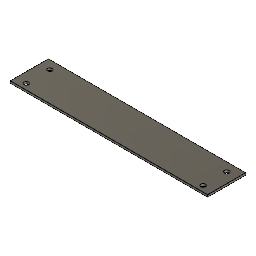
smmb_front-top (Autodesk Fusion 360 design; units mm, degrees)
Autodesk Fusion 360 part; units mm, degrees
sketch "Sketch1" plane through (0, 0, 0) normal (0, 0, 1) x (1, 0, 0)
  line L0 (0, 0) -> (134, 0)
  line L1 (134, 0) -> (134, 26)
  line L2 (134, 26) -> (0, 26)
  line L3 (0, 26) -> (0, 0)
  circle A0 centre (7, 20) radius 1.55
  circle A1 centre (7, 4) radius 1.55
  circle A2 centre (127, 20) radius 1.55
  circle A3 centre (127, 4) radius 1.55
  dimension "d1" = 134
  dimension "d2" = 26
  dimension "d3" = 3.1
  dimension "d4" = 7
  dimension "d5" = 6
  dimension "d6" = 3.1
  dimension "d7" = 7
  dimension "d8" = 4
  dimension "d9" = 3.1
  dimension "d10" = 3.1
  dimension "d11" = 7
  dimension "d12" = 7
  dimension "d13" = 6
  dimension "d14" = 4
  constraint horizontal L0
  constraint vertical L1
  constraint horizontal L2
  constraint vertical L3
  constraint coincident L0.start L3.end
  measures "d1" distance of L0.start L0.end
  measures "d2" distance of L0.start L2.end
  measures "d3" diameter of A0
  measures "d4" distance of L3 A0.centre
  measures "d5" distance of L2 A0.centre
  measures "d6" diameter of A1
  measures "d7" distance of L3 A1.centre
  measures "d8" distance of L0 A1.centre
  measures "d9" diameter of A2
  measures "d10" diameter of A3
  measures "d11" distance of L1 A2.centre
  measures "d12" distance of L1 A3.centre
  measures "d13" distance of L2 A2.centre
  measures "d14" distance of L0 A3.centre
extrude "Extrude1" add sketch "Sketch1" along normal blind 1.5
equation "d6 = d3"
equation "d7 = d4"
equation "d9 = d3"
equation "d10 = d3"
equation "d11 = d4"
equation "d12 = d4"
equation "d13 = d5"
equation "d14 = d8"
